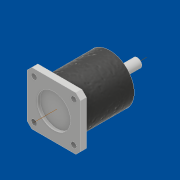
# Autodesk Inventor part: 911-42-reducer-long
Saved by Autodesk Inventor 2018 (Build 220112000, 112)
## iProperties
Created: 2019-12-10
Part Number: 911-42-reducer-long
Material: Generic
Document SubType Name: Modeling
Designer: Bunny320
Density: 1 g/cm^3
Appearance: Default
Author: Bunny320
Autodesk Inventor part; units mm, degrees
ref_plane "YZ Plane" through (0, 0, 0) normal (1, 0, 0) x (0, 1, 0)
ref_plane "XZ Plane" through (0, 0, 0) normal (0, 1, 0) x (-1, 0, 0)
ref_plane "XY Plane" through (0, 0, 0) normal (0, 0, 1) x (1, 0, 0)
sketch "Sketch1" plane through (0, 0, 0) normal (0, 1, 0) x (-1, 0, 0)
  line L0 (-17.5, -17.5) -> (17.5, -17.5)
  line L1 (17.5, -17.5) -> (17.5, 17.5)
  line L2 (17.5, 17.5) -> (-17.5, 17.5)
  line L3 (-17.5, 17.5) -> (-17.5, -17.5)
  line L4 (-17.5, -17.5) -> (17.5, 17.5) construction
  line L5 (17.5, -17.5) -> (-17.5, 17.5) construction
  point P0 (0, 0)
  dimension "d0" = 35
  constraints: 12 end point, 2 midpoint, 2 parallel, 2 perpendicular, 1 horizontal
  measures "d0" distance of L1.end L2.end
extrude "Extrusion1" add sketch "Sketch1" along normal blind 4
sketch "Sketch2" plane through (0, 0, 0) normal (0, 1, 0) x (1, 0, 0)
  circle A0 centre (0, 0) radius 16
  dimension "d3" = 32
  constraints: 1 centre point, 1 coincident
  measures "d3" diameter of A0
extrude "Extrusion2" add sketch "Sketch2" along normal blind 36.8
sketch "Sketch3" plane through (0, 36.8, 0) normal (0, 1, 0) x (1, 0, 0)
  circle A0 centre (0, 0) radius 9.5
  dimension "d6" = 19
  constraints: 1 centre point, 1 coincident
  measures "d6" diameter of A0
extrude "Extrusion3" add sketch "Sketch3" along normal blind 2
sketch "Sketch4" plane through (0, 36.8, 0) normal (0, 1, 0) x (1, 0, 0)
  circle A0 centre (0, 0) radius 3
  dimension "d9" = 6
  constraints: 1 centre point, 1 coincident
  measures "d9" diameter of A0
extrude "Extrusion4" add sketch "Sketch4" along normal blind 18
sketch "Sketch5" plane through (0, 36.8, 0) normal (0, 1, 0) x (1, 0, 0)
  line L0 (24.5, 0) -> (-24.5, 0) projected
  line L1 (0, 24.5) -> (0, -24.5) projected
  point P0 (13, 0)
  dimension "d49" = 13
  constraints: 1 point on line
  measures "d49" distance from line of L1 point (13, 0)
hole "Hole1" at (13, 36.8, 0) direction (0, -1, 0) diameter 2.459 depth 8.8 tip angle 118 thread size "M3x0.5" class "6H" standard "ISO Metric profile"
pattern_circular "Circular Pattern1" count 4 over 360 about axis through (0, -10, 0) along (0, 1, 0) of "Hole1"
chamfer "Chamfer1" distance 3 angle 45 4 edges at (17.5, 2, -17.5) (-17.5, 2, -17.5) (17.5, 2, 17.5) (-17.5, 2, 17.5)
sketch "Sketch7" plane through (0, 0, 0) normal (0, 1, 0) x (-1, 0, 0)
  circle A0 centre (0, 0) radius 11
  dimension "d30" = 22
  constraints: 1 centre point, 1 coincident
  measures "d30" diameter of A0
extrude "Extrusion5" cut sketch "Sketch7" along normal blind 2
sketch "Sketch8" plane through (0, 0, 0) normal (0, 1, 0) x (-1, 0, 0)
  line L0 (13, 13) -> (-13, 13)
  line L1 (-13, 13) -> (-13, -13)
  line L2 (-13, -13) -> (13, -13)
  line L3 (13, -13) -> (13, 13)
  line L4 (13, 13) -> (-13, -13) construction
  line L5 (-13, 13) -> (13, -13) construction
  point P0 (0, 0)
  dimension "d33" = 26
  constraints: 12 end point, 4 coincident, 2 midpoint, 2 parallel, 2 perpendicular, 1 horizontal
  measures "d33" distance of L0.end L1.end
hole "Hole3" at (13, 0, 13) at (-13, 0, 13) at (-13, 0, -13) at (13, 0, -13) direction (0, 1, 0) diameter 3.5 depth 4
sketch "Sketch9" plane through (0, 4, 0) normal (0, 1, 0) x (1, 0, 0)
  circle A0 centre (-13, -13) radius 1.75 projected
  circle A1 centre (-13, 13) radius 1.75 projected
  circle A2 centre (13, 13) radius 1.75 projected
  circle A3 centre (13, -13) radius 1.75 projected
  point P0 (0, 0)
  point P1 (-13.6978, -15.9176)
  point P2 (-15.9176, -13.6978)
  point P3 (13.6978, 15.9176)
  point P4 (15.9176, 13.6978)
  point P5 (14.7912, 17.2088)
  point P6 (-14.7912, -17.2088)
  point P7 (-17.2088, -14.7912)
  point P8 (17.2088, 14.7912)
  constraints: 4 coincident, 2 other
hole "Hole4" at (-13, 4, 13) at (-13, 4, -13) at (13, 4, -13) at (13, 4, 13) direction (0, -1, 0) diameter 6.6 depth 3 tip angle 118
sketch "Sketch10" plane through (0, 54.8, 0) normal (0, 1, 0) x (1, 0, 0)
  line L0 (-4.6716, -4.4668) -> (-2, -4.4668)
  line L1 (-2, -4.4668) -> (-2, 4.6167)
  line L2 (-2, 4.6167) -> (-4.6716, 4.6167)
  line L3 (-4.6716, 4.6167) -> (-4.6716, -4.4668)
  point P0 (0, 0)
  dimension "d53" = 2
  constraints: 8 end point, 2 parallel, 1 horizontal, 1 perpendicular
  measures "d53" distance from line of point (0, 0) L1
extrude "Extrusion6" cut sketch "Sketch10" against normal blind 12
body "Solid1"
